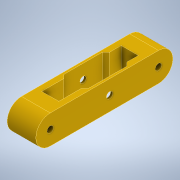
# Autodesk Inventor part: mid
Saved by Autodesk Inventor 2022 (Build 260153000, 153)
## iProperties
Created: 2022-11-09
Part Number: mid
Material: Generic
Document SubType Name: Modeling
Designer: matys
Density: 1 g/cm^3
Appearance: Gold
Author: matys
Autodesk Inventor part; units mm, degrees
ref_plane "YZ Plane" through (0, 0, 0) normal (1, 0, 0) x (0, 1, 0)
ref_plane "XZ Plane" through (0, 0, 0) normal (0, 1, 0) x (-1, 0, 0)
ref_plane "XY Plane" through (0, 0, 0) normal (0, 0, 1) x (1, 0, 0)
sketch "Sketch1" plane through (0, 0, 0) normal (0, 1, 0) x (-1, 0, 0)
  line L0 (0, 0) -> (0, -60)
  line L1 (0, -60) -> (10, -60)
  line L2 (10, -60) -> (10, 0)
  line L3 (10, 0) -> (0, 0)
  line L4 (10, -60) -> (10, -58)
  line L5 (10, -58) -> (0, -58)
  line L6 (10, -58) -> (8, -58)
  line L7 (0, 0) -> (2, 0)
  line L8 (2, 0) -> (2, -2)
  line L9 (2, -2) -> (0, -2)
  line L10 (0, -2) -> (0, 0)
  line L11 (2, -2) -> (8, -2)
  line L12 (8, -2) -> (8, -58)
  line L13 (8, -58) -> (2, -58)
  line L14 (2, -58) -> (2, -2)
  line L15 (10, 0) -> (10, -10)
  line L16 (10, -10) -> (0, -10)
  line L17 (8, -10) -> (8, -18)
  line L18 (8, -18) -> (2, -18)
  line L19 (2, -18) -> (1, -18)
  point P0 (2, -10)
  dimension "d0" = 60
  dimension "d1" = 10
  dimension "d2" = 2
  dimension "d3" = 2
  dimension "d4" = 2
  dimension "d5" = 2
  dimension "d8" = 10
  dimension "d29" = 8
  constraints: 40 end point, 10 point on line, 8 perpendicular, 4 parallel, 2 horizontal, 1 vertical
  measures "d0" distance of L0.start L0.end
  measures "d1" distance of L0.end L1.end
  measures "d2" distance of L1.end L4.end
  measures "d3" distance of L4.end L6.end
  measures "d4" distance of L8.end L9.end
  measures "d5" distance of L7.end L8.end
  measures "d8" distance of L2.end L15.end
  measures "d29" distance of L17.start L17.end
extrude "Extrusion1" add sketch "Sketch1" along normal blind 10 contours L3 L8 L9 L0 | L9 L14 L16 L0 | L3 L2 L16 L12 L11 L8 | L16 L14 L5 L0 | L11 L12 L16 L14 | L5 L2 L1 L0 | L2 L5 L12 L16
fillet "Fillet1" radius 5 2 edges at (-5, 10, 0) (-5, 0, 0)
sketch "Sketch2" plane through (0, 0, -60) normal (1, 0, 0) x (0, 0, -1)
  arc A0 (-55, 10) -> (-55, 0) centre (-55, 5) ccw projected
  line L0 (-55, 10) -> (-55, 0)
  circle A1 centre (-55, 5) radius 1.1
  point P0 (-60, 0)
  dimension "d10" = 2.2
  constraints: 2 end point, 1 centre point, 1 coincident, 1 vertical
  measures "d10" diameter of A1
extrude "Extrusion2" cut sketch "Sketch2" against normal through all contours A1 L0 | L0 A1
sketch "Sketch3" plane through (0, 0, -60) normal (1, 0, 0) x (0, 0, -1)
  circle A0 centre (-55, 5) radius 1.1 projected
  line L0 (-55, 5) -> (-34.322, 5)
  circle A1 centre (-34.322, 5) radius 1.1
  point P0 (-60, 0)
  dimension "d13" = 20.678
  dimension "d53" = 2.2
  constraints: 2 end point, 1 centre point, 1 coincident, 1 horizontal
  measures "d13" distance of L0.start L0.end
  measures "d53" diameter of A1
extrude "Extrusion3" cut sketch "Sketch3" against normal through all contours A1
sketch "Sketch5" plane through (0, 10, 0) normal (0, 1, 0) x (1, 0, 0)
  line L0 (0, 26.778) -> (0, 24.578) projected
  line L1 (0, 25.678) -> (0, 37.678)
  line L2 (0, 37.678) -> (-10, 37.678)
  line L3 (-10, 60) -> (-10, 5) projected
  line L4 (-10, 37.678) -> (-10, 39.678)
  line L5 (-10, 39.678) -> (0, 39.678)
  line L6 (0, 5) -> (0, 60) projected
  line L7 (0, 39.678) -> (0, 41.678)
  line L8 (0, 41.678) -> (-10, 41.678)
  line L9 (-10, 39.678) -> (-10, 41.678)
  line L10 (0, 37.678) -> (0, 47.678)
  line L11 (0, 47.678) -> (-10, 47.678)
  line L12 (-10, 60) -> (-10, 5) projected
  point P0 (0, 0)
  point P1 (0, 41.678)
  dimension "d17" = 12
  dimension "d18" = 2
  dimension "d19" = 2
  dimension "d22" = 10
  constraints: 18 end point, 6 point on line, 5 perpendicular, 2 collinear, 1 midpoint
  measures "d17" distance of L1.start L1.end
  measures "d18" distance of L2.end L4.end
  measures "d19" distance of L5.end L7.end
  measures "d22" distance of L1.end L10.end
extrude "Extrusion4" add sketch "Sketch5" against normal blind 10
sketch "Sketch6" plane through (0, 10, 0) normal (0, 1, 0) x (1, 0, 0)
  line L0 (-10, 60) -> (0, 60)
  line L1 (0, 60) -> (0, 50.678)
  line L2 (0, 50.678) -> (-10, 50.678)
  line L3 (-10, 50.678) -> (-10, 60)
  line L4 (-10, 60) -> (-10, 47.678)
  line L5 (-10, 47.678) -> (0, 47.678)
  line L6 (-2, 47.678) -> (-8, 47.678) projected
  line L7 (0, 47.678) -> (0, 50.678)
  line L8 (0, 5) -> (0, 60) projected
  point P0 (0, 0)
  constraints: 14 end point, 2 collinear, 2 parallel, 1 horizontal, 1 perpendicular, 1 vertical
extrude "Extrusion5" cut sketch "Sketch6" against normal blind 10
sketch "Sketch7" plane through (0, 5, -5) normal (1, 0, 0) x (0, 0, -1)
  line L0 (42.678, 5) -> (0, 5) projected
  circle A0 centre (37.678, 0) radius 1.1
  line L1 (5, 5) -> (32.678, 5) projected
  line L2 (37.678, 5) -> (37.678, -5)
  point P0 (-5, -5)
  point P1 (40.678, 5)
  point P2 (40.678, -5)
  point P3 (45.678, 5)
  constraints: 2 end point, 1 centre point, 1 vertical
extrude "Extrusion6" cut sketch "Sketch7" against normal through all
sketch "Sketch8" plane through (0, 10, 0) normal (0, 1, 0) x (1, 0, 0)
  line L0 (0, 26.778) -> (0, 24.578) projected
  line L1 (0, 25.678) -> (-8, 25.678)
  line L2 (-8, 26.778) -> (-8, 24.578) projected
  line L3 (0, 25.678) -> (0, 17.678)
  line L4 (0, 5) -> (0, 47.678) projected
  line L5 (0, 17.678) -> (-2, 17.678)
  line L6 (-2, 37.678) -> (-2, 10) projected
  line L7 (-2, 17.678) -> (-1, 17.678)
  line L8 (-1, 17.678) -> (-1, 33.678)
  line L9 (-1, 33.678) -> (-2, 33.678)
  line L10 (-2, 33.678) -> (-9, 33.678)
  line L11 (-9, 33.678) -> (-9, 17.678)
  line L12 (-9, 17.678) -> (-2, 17.678)
  line L13 (-9, 33.678) -> (-9.25, 33.678)
  line L14 (-9.25, 33.678) -> (-9.25, 17.678)
  line L15 (-9.25, 17.678) -> (-9, 17.678)
  line L16 (-1, 17.678) -> (-0.75, 17.678)
  line L17 (-0.75, 17.678) -> (-0.75, 33.678)
  line L18 (-0.75, 33.678) -> (-1, 33.678)
  point P0 (0, 0)
  point P1 (0, 45.678)
  point P2 (0, 50.678)
  dimension "d30" = 8
  dimension "d31" = 16
  dimension "d32" = 7
  dimension "d50" = 0.25
  dimension "d51" = 0.25
  constraints: 30 end point, 6 perpendicular, 6 point on line, 3 midpoint, 2 horizontal, 2 parallel
  measures "d30" distance of L1.start L3.end
  measures "d31" distance of L7.end L8.end
  measures "d32" distance of L9.end L10.end
  measures "d50" distance of L10.end L13.end
  measures "d51" distance of L7.end L16.end
extrude "Extrusion7" cut sketch "Sketch8" against normal blind 10 contours L17 L5 L8 L1 | L1 L8 L18 L17 | L8 L5 L6 L1 | L1 L6 L9 L8 | L6 L12 L11 L10 | L11 L15 L14 L13
fillet "Fillet3" radius 5 2 edges at (-5, 10, -47.678) (-5, 0, -47.678)
chamfer "Chamfer2" distance 1.25 angle 45 4 edges at (-9.25, 5, -17.678) (-9.25, 5, -33.678) (-0.75, 5, -17.678) (-0.75, 5, -33.678)
body "Solid1"
